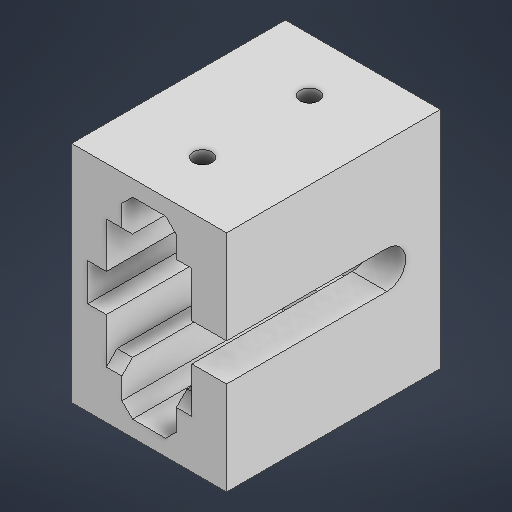
# Autodesk Inventor part: tensionerholder
Saved by Autodesk Inventor 2025.1 (Build 291241000, 241)
## iProperties
Created: 2025-02-02
Part Number: tensionerholder
Material: Generic
Document SubType Name: Modeling
Designer: jerem
Density: 1 g/cm^3
Appearance: Default
Author: jerem
## iProperties of the stored document tensionerholder_3DPrint.ipt
Created: 2025-02-02
Part Number: tensionerholder_3DPrint
Material: Generic
Document SubType Name: Modeling
Designer: jerem
Density: 1 g/cm^3
Appearance: Default
Author: jerem
Autodesk Inventor part; units mm, degrees
ref_plane "YZ Plane" through (0, 0, 0) normal (1, 0, 0) x (0, 1, 0)
ref_plane "XZ Plane" through (0, 0, 0) normal (0, 1, 0) x (-1, 0, 0)
ref_plane "XY Plane" through (0, 0, 0) normal (0, 0, 1) x (1, 0, 0)
sketch "Sketch1" plane through (0, 0, 0) normal (0, 1, 0) x (-1, 0, 0)
  line L0 (8, 0) -> (8, -35)
  line L1 (8, -35) -> (-8, -35)
  line L2 (-8, -35) -> (-8, 0)
  line L3 (-8, 0) -> (0, 0)
  line L4 (0, 0) -> (8, 0)
  line L5 (-8, 0) -> (-14.5, 0)
  line L6 (-14.5, 0) -> (-14.5, -40)
  line L7 (-14.5, -40) -> (14.5, -40)
  line L8 (14.5, -40) -> (14.5, 0)
  line L9 (14.5, 0) -> (8, 0)
  line L10 (5.1, 0) -> (5.1, -30)
  line L11 (5.1, -30) -> (-5.1, -30)
  line L12 (-5.1, -30) -> (-5.1, 0)
  line L13 (-5.1, -30) -> (-8, -30) construction
  line L14 (5.1, -30) -> (8, -30) construction
  dimension "d2" = 5
  dimension "d17" = 5
  dimension "d26" = 29
  dimension "d27" = 10.2
  dimension "d28" = 16
  dimension "d29" = 40
  constraints: 30 end point, 9 perpendicular, 6 point on line, 4 collinear, 2 horizontal, 2 vertical
  measures "d2" distance between parallel lines of L7 L1
  measures "d17" distance between parallel lines of L1 L11
  measures "d26" distance between parallel lines of L6 L8
  measures "d27" distance between parallel lines of L12 L10
  measures "d28" distance between parallel lines of L0 L2
  measures "d29" distance from line of L8.end L7
extrude "Extrusion1" add sketch "Sketch1" along normal blind 42 contours L9 L8 L7 L6 L5 L2 L1 L0
sketch "Sketch2" plane through (14.5, 0, 0) normal (1, 0, 0) x (0, 0, -1)
  line L0 (0, 0) -> (40, 0) projected
  line L1 (40, 0) -> (40, 42) projected
  line L2 (0, 42) -> (40, 42) projected
  line L3 (0, 0) -> (0, 42) projected
  line L4 (0, 21) -> (0, 21) construction
  circle A0 centre (0, 21) radius 3.5
  line L5 (0, 21) -> (30, 21) construction
  circle A1 centre (30, 21) radius 3.5
  line L6 (0, 24.5) -> (30, 24.5)
  line L7 (30, 17.5) -> (0, 17.5)
  line L8 (0, 0) -> (0, 42) projected
  point P0 (0, 21)
  dimension "d6" = 7
  dimension "d8" = 0
  dimension "d40" = 30
  constraints: 8 end point, 4 point on circle, 4 tangent, 2 centre point, 2 coincident, 2 horizontal, 2 midpoint, 1 equal radius
  measures "d6" diameter of A0
  measures "d8" distance from line of L3 L4.end
  measures "d40" distance of point (0, 21) L5.end
extrude "Extrusion2" cut sketch "Sketch2" against normal blind 26 contours A0 L3 | L3 A0 | A0 L6 A1 L7 | A1
sketch "Sketch3" plane through (14.5, 0, -40) normal (0, 0, -1) x (-1, 0, 0)
  line L0 (0, 0) -> (29, 0) projected
  line L1 (29, 0) -> (29, 42) projected
  line L2 (0, 42) -> (29, 42) projected
  line L3 (0, 0) -> (0, 42) projected
  line L4 (29, 0) -> (29, 42) construction
  line L5 (29, 21) -> (14.5, 21) construction
  line L6 (14.5, 21) -> (14.5, 0) construction
  circle A0 centre (14.5, 21) radius 1.8
  dimension "d11" = 3.6
  constraints: 4 end point, 2 perpendicular, 1 centre point, 1 coincident, 1 midpoint
  measures "d11" diameter of A0
extrude "Extrusion3" cut sketch "Sketch3" against normal blind 10 contours A0
extrude "Extrusion4" add sketch "Sketch1" along normal blind 11 contours L0 L1 L2 L3 L12 L11 L10 L4
extrude "Extrusion5" add sketch "Sketch1" along normal blind 3 contours L10 L11 L12 L3 L4
chamfer "Chamfer1" distance 2 angle 45 3 edges at (-5.1, 3, -15) (0, 3, -30) (5.1, 3, -15)
chamfer "Chamfer2" distance 2 angle 45 2 edges at (-6.55, 11, 0) (6.55, 11, 0)
ref_plane "Work Plane1" through (0, 21, 0) normal (0, 1, 0) x (1, 0, 0)
mirror "Mirror1" about plane through (0, 21, 0) normal (0, 1, 0) of "Extrusion4", "Extrusion5", "Chamfer1", "Chamfer2"
sketch "Sketch4" plane through (0, 42, 0) normal (0, 1, 0) x (1, 0, 0)
  line L0 (-14.5, 0) -> (14.5, 0) projected
  line L1 (14.5, 0) -> (14.5, 40) projected
  line L2 (14.5, 40) -> (-14.5, 40) projected
  line L3 (-14.5, 40) -> (-14.5, 0) projected
  line L4 (0, 0) -> (0, 10) construction
  circle A0 centre (0, 10) radius 1.75
  line L5 (0, 10) -> (0, 30) construction
  circle A1 centre (0, 30) radius 1.75
  dimension "d30" = 3.5
  dimension "d31" = 10
  dimension "d32" = 20
  constraints: 4 end point, 2 centre point, 2 coincident, 2 vertical, 1 equal radius
  measures "d30" diameter of A0
  measures "d31" distance from line of L5.end L2
  measures "d32" distance of L5.start L5.end
extrude "Extrusion6" cut sketch "Sketch4" against normal up to surface (3 mm away) contours A0 | A1
sketch "Sketch5" plane through (14.5, 0, -40) normal (0, 0, -1) x (-1, 0, 0)
  circle A0 centre (14.5, 21) radius 1.8 projected
  line L0 (0, 0) -> (29, 0) projected
  line L1 (29, 0) -> (29, 42) projected
  line L2 (0, 42) -> (29, 42) projected
  line L3 (0, 0) -> (0, 42) projected
  line L4 (14.5, 0) -> (14.5, 8) construction
  line L5 (14.5, 8) -> (22, 8) construction
  line L6 (14.5, 8) -> (7, 8) construction
  circle A1 centre (7, 8) radius 1.75
  circle A2 centre (22, 8) radius 1.75
  dimension "d35" = 8
  dimension "d36" = 3.5
  dimension "d39" = 15
  constraints: 6 end point, 2 centre point, 2 coincident, 1 collinear, 1 equal radius, 1 horizontal, 1 perpendicular, 1 vertical
  measures "d35" distance of L4.start L4.end
  measures "d36" diameter of A1
  measures "d39" distance of L5.end L6.end
extrude "Extrusion7" cut sketch "Sketch5" against normal blind 6 contours A1 | A2
mirror "Mirror2" about plane through (0, 21, 0) normal (0, 1, 0) of "Extrusion6"
body "Solid1"
